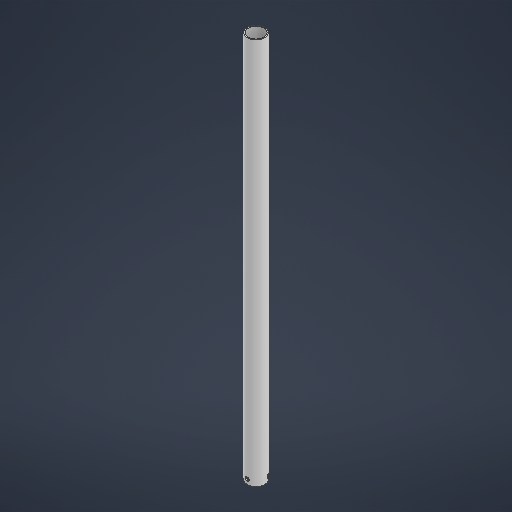
# Autodesk Inventor part: Pieza38
Saved by Autodesk Inventor 2026.2 (Build 302298000, 298)
## iProperties
Created: 2026-01-02
Part Number: Pieza38
Material: Genérico
Document SubType Name: Modeling
Designer: vicho
Density: 1 g/cm^3
Appearance: Valor por defecto
Author: vicho
Autodesk Inventor part; units mm, degrees
ref_plane "XZ Plane" through (0, 0, 0) normal (0, 1, 0) x (-1, 0, 0)
sketch "Boceto1" plane through (0, 0, 0) normal (0, 1, 0) x (-1, 0, 0)
  circle A0 centre (0, 0) radius 18.5
  dimension "d0" = 37
  constraints: 1 centre point, 1 coincident
  measures "d0" diameter of A0
extrude "Extrusión1" add sketch "Boceto1" along normal blind 805
shell "Vaciado1" thickness 2 removed faces 2 at (3.5031, 0, 5.0751) at (3.5031, 805, 5.0751)
ref_plane "Plano de trabajo1" through (0, 0, 18.5) normal (0, 0, 1) x (1, 0, 0)
ref_plane "Plano de trabajo2" through (18.5, 0, 0) normal (1, 0, 0) x (0, 1, 0)
sketch "Boceto4" plane through (0, 0, 18.5) normal (0, 0, 1) x (1, 0, 0)
  line L0 (0, 18.0734) -> (0, -36.4146) construction
  line L1 (47.7272, 0) -> (-52.5468, 0) construction
  circle A0 centre (0, 10) radius 4
  point P0 (0, 0)
  dimension "d14" = 8
  dimension "d15" = 10
  constraints: 4 end point, 3 point on line, 1 centre point, 1 horizontal, 1 vertical
  measures "d14" diameter of A0
  measures "d15" distance from line of L1 A0.centre
extrude "Extrusión4" cut sketch "Boceto4" against normal blind 10
pattern_circular "Patrón circular1" count 3 over 360 about axis through (0, 0, 0) along (0, 1, 0) of "Extrusión4"
